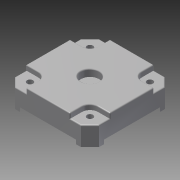
# Autodesk Inventor part: stepper_front
Saved by Autodesk Inventor 2013 (Build 170138000, 138)
## iProperties
Created: 2011-05-14
Part Number: stepper_front
Document SubType Name: Modeling
Designer: Noa Izumi
Material: Default
Density: 1 g/cm^3
Control State: 0
Master: False
Checked Out: False
Shininess: 50.0
Density: 0.0
Volumn: 0.0
Area: 0.0
PropertySet Name: Model Information
Author: Noa Izumi
Autodesk Inventor part; units mm, degrees
ref_plane "YZ Plane" through (0, 0, 0) normal (1, 0, 0) x (0, 1, 0)
ref_plane "XZ Plane" through (0, 0, 0) normal (0, 1, 0) x (-1, 0, 0)
ref_plane "XY Plane" through (0, 0, 0) normal (0, 0, 1) x (1, 0, 0)
sketch "Sketch1" plane through (0, 0, 0) normal (0, 0, 1) x (1, 0, 0)
  line L0 (0, 0) -> (42, 0)
  line L1 (42, 0) -> (42, 42)
  line L2 (42, 42) -> (0, 42)
  line L3 (0, 42) -> (0, 0)
  dimension "d0" = 42
  dimension "d1" = 42
  constraints: 8 end point, 2 parallel, 1 horizontal, 1 perpendicular
  measures "d0" distance of L2.end L0.start
  measures "d1" distance of L0.start L0.end
extrude "Extrusion1" add sketch "Sketch1" along normal blind 9.5
chamfer "Chamfer1" distance 4.5 angle 45 4 edges at (0, 0, 4.75) (42, 0, 4.75) (42, 42, 4.75) (0, 42, 4.75)
sketch "Sketch6" plane through (0, 0, 0) normal (0, 0, -1) x (-1, 0, 0)
  line L0 (-42, 4.5) -> (-42, 37.5) projected
  line L1 (-4.5, 0) -> (-37.5, 0) projected
  circle A0 centre (-21, 21) radius 25.25
  dimension "d37" = 50.5
  dimension "d38" = 21
  dimension "d39" = 21
  constraints: 1 centre point
  measures "d37" diameter of A0
  measures "d38" distance from line of L0 A0.centre
  measures "d39" distance from line of L1 A0.centre
extrude "Extrusion5" cut sketch "Sketch6" against normal blind 2
sketch "Sketch2" plane through (0, 0, 9.5) normal (0, 0, 1) x (1, 0, 0)
  line L0 (4.5, 42) -> (37.5, 42) projected
  line L1 (0, 4.5) -> (0, 37.5) projected
  line L2 (37.5, 0) -> (4.5, 0) projected
  line L3 (42, 37.5) -> (42, 4.5) projected
  line L4 (10, 0) -> (10, 6)
  line L5 (10, 36) -> (10, 42)
  line L6 (0, 32) -> (6, 32)
  line L7 (36, 32) -> (42, 32)
  line L8 (0, 10) -> (6, 10)
  line L9 (36, 10) -> (42, 10)
  line L10 (32, 42) -> (32, 36)
  line L11 (32, 6) -> (32, 0)
  arc A0 (6, 32) -> (10, 36) centre (6, 36) ccw
  arc A1 (32, 36) -> (36, 32) centre (36, 36) ccw
  arc A2 (36, 10) -> (32, 6) centre (36, 6) ccw
  arc A3 (10, 6) -> (6, 10) centre (6, 6) ccw
  dimension "d10" = 4
  constraints: 16 end point, 10 parallel, 8 point on circle, 8 point on line, 8 tangent, 4 centre point, 4 perpendicular, 3 equal radius
  measures "d10" radius of A0
extrude "Extrusion6" add sketch "Sketch2" along normal blind 2.5
fillet "Fillet3" radius 0.5 35 edges at (2.25, 2.25, 9.5) (7.25, 0, 9.5) (0, 7.25, 9.5) (34.75, 0, 9.5) (39.75, 2.25, 9.5) (42, 7.25, 9.5) (42, 34.75, 9.5) (34.75, 42, 9.5) (39.75, 39.75, 9.5) (0, 34.75, 9.5) (2.25, 39.75, 9.5) (7.25, 42, 9.5) (0, 21, 12) (42, 21, 12) (3, 10, 12) (8.8284, 8.8284, 12) (10, 3, 12) (21, 0, 12) (32, 3, 12) (33.1716, 8.8284, 12) (39, 10, 12) (33.1716, 33.1716, 12) (39, 32, 12) (32, 39, 12) (8.8284, 33.1716, 12) (10, 39, 12) (3, 32, 12) (21, 42, 12) (10, 0, 10.75) (32, 0, 10.75) (42, 10, 10.75) (42, 32, 10.75) (32, 42, 10.75) (10, 42, 10.75) (0, 32, 10.75)
sketch "Sketch7" plane through (0, 0, 12) normal (0, 0, 1) x (1, 0, 0)
  circle A0 centre (21, 21) radius 4.5
  line L0 (31.5, 42) -> (10.5, 42) projected
  line L1 (0, 31.5) -> (0, 10) projected
  dimension "d45" = 9
  dimension "d46" = 21
  dimension "d47" = 21
  constraints: 1 centre point
  measures "d45" diameter of A0
  measures "d46" distance from line of L0 A0.centre
  measures "d47" distance from line of L1 A0.centre
extrude "Extrusion7" cut sketch "Sketch7" against normal blind 3.5
fillet "Fillet4" radius 0.5 1 edges at (16.5, 21, 12)
sketch "Sketch8" plane through (0, 0, 9.5) normal (0, 0, 1) x (1, 0, 0)
  arc A0 (10, 6) -> (6, 10) centre (6, 6) ccw projected
  point P0 (36, 6)
  point P1 (6, 36)
  point P2 (36, 36)
  dimension "d51" = 30
  dimension "d52" = 30
  constraints: 1 coincident
  measures "d51" distance of point (6, 36) A0.centre
  measures "d52" distance of point (36, 6) A0.centre
hole "Hole2" at (6, 6, 9.5) at (36, 6, 9.5) at (6, 36, 9.5) at (36, 36, 9.5) direction (0, 0, -1) diameter 3 depth 5
